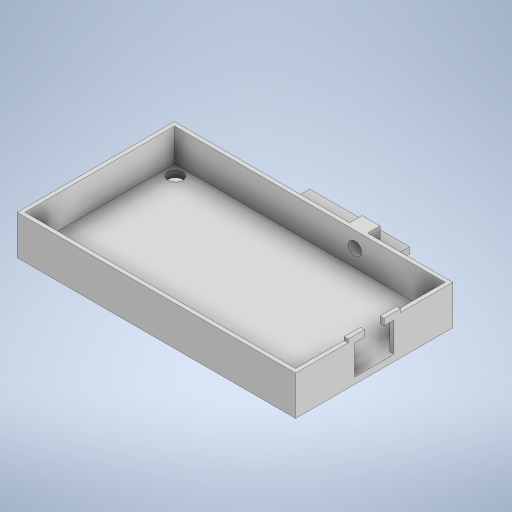
# Autodesk Inventor part: prent1
Saved by Autodesk Inventor 2023 (Build 270158000, 158)
## iProperties
Created: 2023-01-05
Part Number: prent1
Material: Ogólny
Document SubType Name: Modeling
Designer: User
Density: 1 g/cm^3
Appearance: Domyślna
Author: User
Autodesk Inventor part; units mm, degrees
ref_plane "YZ Plane" through (0, 0, 0) normal (1, 0, 0) x (0, 1, 0)
ref_plane "XZ Plane" through (0, 0, 0) normal (0, 1, 0) x (-1, 0, 0)
ref_plane "XY Plane" through (0, 0, 0) normal (0, 0, 1) x (1, 0, 0)
sketch "Szkic2" plane through (0, 0, 0) normal (0, 1, 0) x (-1, 0, 0)
  line L0 (42.5, 24) -> (-42.5, 24)
  line L1 (-42.5, 24) -> (-42.5, -24)
  line L2 (-42.5, -24) -> (42.5, -24)
  line L3 (42.5, -24) -> (42.5, 24)
  line L4 (0, 91.0722) -> (0, -100.1143)
  line L5 (-78.4738, 0) -> (170.7955, 0)
  circle A0 centre (37.932, 19.715) radius 2.25
  circle A1 centre (37.932, -19.715) radius 2.25
  circle A2 centre (-37.932, 19.715) radius 2.25
  circle A3 centre (-37.932, -19.715) radius 2.25
  point P0 (0, 0)
  dimension "d7" = 48
  dimension "d8" = 85
  dimension "d14" = 4.5
  dimension "d16" = 39.43
  dimension "d18" = 24
  dimension "d21" = 75.864
  dimension "d22" = 42.5
  constraints: 12 end point, 4 centre point, 3 horizontal, 3 symmetric about line, 2 parallel, 2 vertical, 1 perpendicular, 3 other
  measures "d7" distance of L2.end L0.start
  measures "d8" distance of L0.start L0.end
  measures "d14" diameter of A0
  measures "d16" distance of A1.centre A0.centre
  measures "d18" distance between parallel lines of L5 L0
  measures "d21" distance of A2.centre A0.centre
  measures "d22" distance between parallel lines of L4 L3
extrude "Wyciągnięcie proste2" add sketch "Szkic2" along normal blind 2
sketch "Szkic3" plane through (0, 2, 0) normal (0, 1, 0) x (1, 0, 0)
  line L0 (-42.5, -24) -> (42.5, -24) projected
  line L1 (42.5, -24) -> (42.5, 24) projected
  line L2 (41.3, -24) -> (42.5, -24)
  line L3 (42.5, -24) -> (42.5, 24)
  line L4 (42.5, 24) -> (41.3, 24)
  line L5 (41.3, 24) -> (41.3, -24)
  line L6 (-42.5, 24) -> (-42.5, -24) projected
  line L7 (42.5, -24) -> (-42.5, -24)
  line L8 (-42.5, -24) -> (-42.5, -22.8)
  line L9 (-42.5, -22.8) -> (42.5, -22.8)
  line L10 (42.5, -22.8) -> (42.5, -24)
  line L11 (42.5, 24) -> (-42.5, 24)
  line L12 (-42.5, 24) -> (-42.5, 22.8)
  line L13 (-42.5, 22.8) -> (42.5, 22.8)
  line L14 (42.5, 22.8) -> (42.5, 24)
  line L15 (42.5, 24) -> (-42.5, 24) projected
  line L16 (-42.5, -24) -> (-41.3, -24)
  line L17 (-41.3, -24) -> (-41.3, 24)
  line L18 (-41.3, 24) -> (-42.5, 24)
  line L19 (-42.5, 24) -> (-42.5, -24)
  line L20 (42.5, -6) -> (41.3, -6)
  line L21 (41.3, -6) -> (41.3, 6)
  line L22 (41.3, 6) -> (42.5, 6)
  line L23 (36.3786, 0) -> (45.7918, 0)
  point P0 (0, 0)
  point P1 (41.3, -22.8)
  point P2 (-41.3, -22.8)
  point P3 (-41.3, 22.8)
  point P4 (41.3, 22.8)
  dimension "d25" = 1.2
  dimension "d26" = 1.2
  dimension "d27" = 1.2
  dimension "d28" = 1.2
  dimension "d29" = 12
  dimension "d30" = 6
  constraints: 40 end point, 9 parallel, 7 horizontal, 6 point on line, 5 perpendicular
  measures "d25" distance between parallel lines of L0 L9
  measures "d26" distance between parallel lines of L1 L5
  measures "d27" distance between parallel lines of L17 L19
  measures "d28" distance between parallel lines of L13 L11
  measures "d29" distance between parallel lines of L22 L20
  measures "d30" distance between parallel lines of L23 L20
extrude "Wyciągnięcie proste3" add sketch "Szkic3" along normal blind 10 contours L6 L9 L17 L0 | L17 L9 L5 L0 | L6 L13 L17 L9 | L5 L9 L1 L0 | L6 L11 L17 L13 | L5 L20 L1 L9 | L17 L11 L5 L13 | L13 L1 L22 L5 | L5 L4 L1 L13
sketch "Szkic5" plane through (0, 12, 0) normal (0, 1, 0) x (1, 0, 0)
  line L0 (41.3, -6) -> (41.3, -22.8) projected
  line L1 (42.5, -6) -> (42.5, 6) projected
  line L2 (41.3, -8) -> (42.5, -8)
  line L3 (42.5, -8) -> (42.5, -3)
  line L4 (42.5, -3) -> (41.3, -3)
  line L5 (41.3, -3) -> (41.3, -8)
  line L6 (34.6755, 0) -> (49.4443, 0)
  line L7 (40.0187, -6) -> (43.7777, -6)
  line L8 (41.3, 8) -> (42.5, 8)
  line L9 (42.5, 8) -> (42.5, 3)
  line L10 (42.5, 3) -> (41.3, 3)
  line L11 (41.3, 3) -> (41.3, 8)
  line L12 (40.0187, 6) -> (43.7777, 6)
  point P0 (0, 0)
  point P1 (41.3, 6)
  dimension "d33" = 5
  dimension "d34" = 2
  constraints: 22 end point, 6 symmetric about line, 5 horizontal, 2 parallel, 2 point on line, 1 perpendicular
  measures "d33" distance of L4.end L2.start
  measures "d34" distance between parallel lines of L7 L2
extrude "Wyciągnięcie proste4" add sketch "Szkic5" along normal blind 1 contours L7 L3 L2 L0 | L12 L11 L8 L9
extrude "Wyciągnięcie proste5" add sketch "Szkic5" along normal mid plane 2 contours L5 L4 L1 L7 | L10 L11 L12 L1
sketch "Szkic6" plane through (42.5, 0, -24) normal (0, 0, -1) x (-1, 0, 0)
  line L0 (83.8, 12) -> (1.2, 12) projected
  line L1 (26, 12) -> (26, 0)
  line L2 (31.5, 12) -> (31.5, 0)
  line L3 (53.5, 12) -> (53.5, 0)
  line L4 (0, 0) -> (85, 0) projected
  line L5 (56.5, 12) -> (56.5, 0)
  line L6 (0, 0) -> (0, 12) projected
  circle A0 centre (28.6456, 7.207) radius 1.5875
  line L7 (1.2, 2) -> (83.8, 2) projected
  line L8 (26, 2) -> (56.5, 2)
  point P0 (42.5, 0)
  dimension "d39" = 5.5
  dimension "d40" = 22
  dimension "d41" = 3
  dimension "d42" = 31.5
  dimension "d43" = 3.175
  dimension "d55" = 5.207
  constraints: 11 point on line, 10 end point, 3 vertical, 1 centre point, 1 perpendicular
  measures "d39" distance between parallel lines of L2 L1
  measures "d40" distance between parallel lines of L3 L2
  measures "d41" distance between parallel lines of L5 L3
  measures "d42" distance between parallel lines of L2 L6
  measures "d43" diameter of A0
  measures "d55" distance from line of L7 A0.centre
sketch "Szkic8" plane through (0, 0, 0) normal (0, -1, 0) x (1, 0, 0)
  line L0 (42.5, -24) -> (-42.5, -24) projected
  line L1 (20.6822, -24) -> (-15.9857, -24)
  line L2 (-15.9857, -24) -> (-15.9857, -43.1071)
  line L3 (-15.9857, -43.1071) -> (20.6822, -43.1071)
  line L4 (20.6822, -43.1071) -> (20.6822, -24)
  line L5 (16.5, -24) -> (11, -24)
  line L6 (11, -24) -> (11, -36.8)
  line L7 (11, -36.8) -> (16.5, -36.8)
  line L8 (16.5, -36.8) -> (16.5, -24)
  line L9 (11, -24) -> (-11, -24)
  line L10 (-11, -24) -> (-11, -36.8)
  line L11 (-11, -36.8) -> (11, -36.8)
  line L12 (11, -36.8) -> (11, -24)
  line L13 (-11, -24) -> (-14, -24)
  line L14 (-14, -24) -> (-14, -36.8)
  line L15 (-14, -36.8) -> (-11, -36.8)
  line L16 (-11, -36.8) -> (-11, -24)
  line L17 (16.5, -27.8) -> (-14, -27.8)
  point P0 (0, 0)
  point P1 (11, -27.8)
  dimension "d45" = 5.5
  dimension "d46" = 22
  dimension "d47" = 3
  dimension "d48" = 31.5
  dimension "d49" = 3.8
  dimension "d50" = 9
  constraints: 34 end point, 8 parallel, 5 perpendicular, 4 horizontal, 4 point on line
  measures "d45" distance between parallel lines of L6 L8
  measures "d46" distance of L6.end L10.end
  measures "d47" distance of L14.end L15.end
  measures "d48" distance from line of L0.start L6
  measures "d49" distance between parallel lines of L17 L0
  measures "d50" distance of L7.end L17.start
extrude "Wyciągnięcie proste6" add sketch "Szkic8" against normal blind 2 contours L6 L17 L10 L0 | L8 L7 L6 L17 | L10 L17 L14 L0 | L6 L11 L10 L17 | L10 L15 L14 L17
extrude "Wyciągnięcie proste7" add sketch "Szkic8" against normal blind 12 contours L8 L17 L6 L0
hole "Otwór1" at (13.8544, 7.207, -24) direction (0, 0, -1) diameter 4 depth 4 start extended yes
